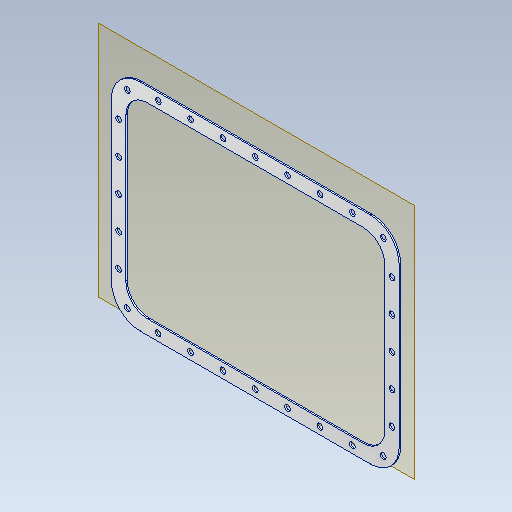
# Autodesk Inventor part: Прокладка крышки фонаря 1_CPY
Saved by Autodesk Inventor 2021 (Build 250183000, 183)
## iProperties
Created: 2020-12-10
Part Number: Прокладка крышки фонаря 1_CPY
Material: Алюминий 6061
Document SubType Name: Modeling
Designer: Тимоха
Mass: 131.715 g
Surface Area: 552.304 cm^2
Volume: 48.7834 cm^3
Density: 2.7 g/cm^3
Appearance: Алюминий — плоский
Author: Тимоха
Autodesk Inventor part; units mm, degrees
ref_plane "YZ Plane" through (0, 0, 0) normal (1, 0, 0) x (0, 1, 0)
ref_plane "XZ Plane" through (0, 0, 0) normal (0, 1, 0) x (-1, 0, 0)
ref_plane "XY Plane" through (0, 0, 0) normal (0, 0, 1) x (1, 0, 0)
ref_plane "РабПлоскость1" through (0, 0, 0) normal (0, 0, 1) x (1, 0, 0)
sketch "Эскиз1" plane through (0, 0, 0) normal (0, 0, 1) x (1, 0, 0)
  circle A0 centre (190, 19.9968) radius 4 projected
  circle A1 centre (190, 64.9937) radius 4 projected
  circle A2 centre (177.9182, 106.4529) radius 4 projected
  circle A3 centre (134.9905, 115) radius 4 projected
  circle A4 centre (89.9937, 115) radius 4 projected
  circle A5 centre (44.9968, 115) radius 4 projected
  circle A6 centre (0, 115) radius 4 projected
  circle A7 centre (-44.9968, 115) radius 4 projected
  circle A8 centre (-89.9937, 115) radius 4 projected
  circle A9 centre (-134.9905, 115) radius 4 projected
  circle A10 centre (-177.9182, 106.4529) radius 4 projected
  circle A11 centre (-190, 64.9937) radius 4 projected
  circle A12 centre (-190, 19.9968) radius 4 projected
  circle A13 centre (-190, -25) radius 4 projected
  circle A14 centre (-190, -69.9968) radius 4 projected
  circle A15 centre (-190, -114.9937) radius 4 projected
  circle A16 centre (-177.9182, -156.4529) radius 4 projected
  circle A17 centre (-134.9905, -165) radius 4 projected
  circle A18 centre (-89.9937, -165) radius 4 projected
  circle A19 centre (-44.9968, -165) radius 4 projected
  circle A20 centre (0, -165) radius 4 projected
  circle A21 centre (44.9968, -165) radius 4 projected
  circle A22 centre (89.9937, -165) radius 4 projected
  circle A23 centre (134.9905, -165) radius 4 projected
  circle A24 centre (177.9182, -156.4529) radius 4 projected
  circle A25 centre (190, -114.9937) radius 4 projected
  circle A26 centre (190, -69.9968) radius 4 projected
  circle A27 centre (190, -25) radius 4 projected
  line L0 (-200, -135) -> (-200, 85) projected
  arc A28 (-200, -135) -> (-160, -175) centre (-160, -135) ccw projected
  line L1 (160, -175) -> (-160, -175) projected
  arc A29 (160, -175) -> (200, -135) centre (160, -135) ccw projected
  line L2 (200, 85) -> (200, -135) projected
  arc A30 (200, 85) -> (160, 125) centre (160, 85) ccw projected
  line L3 (-160, 125) -> (160, 125) projected
  arc A31 (-160, 125) -> (-200, 85) centre (-160, 85) ccw projected
  line L4 (-150, -155) -> (150, -155) projected
  arc A32 (-180, -125) -> (-150, -155) centre (-150, -125) ccw projected
  line L5 (-180, 75) -> (-180, -125) projected
  arc A33 (-150, 105) -> (-180, 75) centre (-150, 75) ccw projected
  line L6 (150, 105) -> (-150, 105) projected
  arc A34 (180, 75) -> (150, 105) centre (150, 75) ccw projected
  line L7 (180, -125) -> (180, 75) projected
  arc A35 (150, -155) -> (180, -125) centre (150, -125) ccw projected
  point P0 (0, 0)
extrude "Выдавливание1" add sketch "Эскиз1" along normal blind 2
